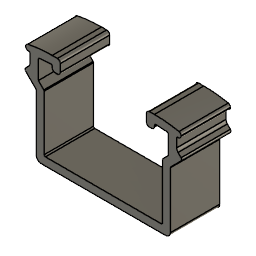
AdaptadorCristal9mm (Autodesk Fusion 360 design; units mm, degrees)
part number: 2025-12-28-14-56-03-854
Autodesk Fusion 360 part; units mm, degrees
sketch "Boceto1" plane through (0, 0, 0) normal (0, 1, 0) x (1, 0, 0)
  line L0 (2.05, 0) -> (0, 0) construction
  line L1 (3.05, 0) -> (15.65, 0)
  line L2 (2.05, -12.3964) -> (2.05, -1)
  arc A0 (3.05, 0) -> (2.05, -1) centre (3.05, -1) ccw
  line L3 (3.6762, -10.8738) -> (3.6762, -1.8762)
  line L4 (3.9262, -1.6262) -> (15.65, -1.6262)
  arc A1 (3.9262, -1.6262) -> (3.6762, -1.8762) centre (3.9262, -1.8762) ccw
  line L5 (1.9767, -12.5732) -> (-0.0927, -14.6402)
  line L6 (0.5221, -15.8217) -> (-0.093, -15.2059)
  arc A2 (-0.0927, -14.6402) -> (-0.093, -15.2059) centre (0.19, -14.9232) ccw
  line L7 (0.8, -16.4931) -> (0.8, -18.25)
  line L8 (0.6, -18.45) -> (0.45, -18.45)
  arc A3 (0.8, -16.4931) -> (0.5221, -15.8217) centre (-0.15, -16.4931) ccw
  arc A4 (0.6, -18.45) -> (0.8, -18.25) centre (0.6, -18.25) ccw
  line L9 (3.6762, -10.8738) -> (3.6762, -13.0203)
  line L10 (2.5, -14.3) -> (3.6029, -13.1971)
  line L11 (2.5, -14.3) -> (2.5, -18.0672)
  line L12 (2.7322, -18.3166) -> (5.0322, -18.4809)
  line L13 (5.3, -18.2315) -> (5.3, -17.95)
  line L14 (5.9, -17.35) -> (6.35, -17.35)
  line L15 (6.95, -17.95) -> (6.95, -19.5)
  line L16 (6.35, -20.1) -> (5.3, -20.1)
  line L17 (-0.1, -19) -> (-0.1, -19.0559)
  arc A5 (0.3391, -19.5946) -> (5.3, -20.1) centre (5.3, 4.5) ccw
  arc A6 (-0.1, -19.0559) -> (0.3391, -19.5946) centre (0.45, -19.0559) ccw
  arc A7 (0.45, -18.45) -> (-0.1, -19) centre (0.45, -19) ccw
  arc A8 (6.35, -20.1) -> (6.95, -19.5) centre (6.35, -19.5) ccw
  arc A9 (6.95, -17.95) -> (6.35, -17.35) centre (6.35, -17.95) ccw
  arc A10 (5.9, -17.35) -> (5.3, -17.95) centre (5.9, -17.95) ccw
  arc A11 (5.0322, -18.4809) -> (5.3, -18.2315) centre (5.05, -18.2315) ccw
  arc A12 (2.5, -18.0672) -> (2.7322, -18.3166) centre (2.75, -18.0672) ccw
  arc A13 (3.6029, -13.1971) -> (3.6762, -13.0203) centre (3.4262, -13.0203) ccw
  arc A14 (1.9767, -12.5732) -> (2.05, -12.3964) centre (1.8, -12.3964) ccw
  line L18 (15.65, 0) -> (15.65, -24.4844) construction
  line L19 (28.8, -14.3) -> (27.6971, -13.1971)
  line L20 (27.6238, -10.8738) -> (27.6238, -13.0203)
  arc A15 (24.35, -19.5) -> (24.95, -20.1) centre (24.95, -19.5) ccw
  line L21 (30.7, -18.45) -> (30.85, -18.45)
  line L22 (29.25, -12.3964) -> (29.25, -1)
  line L23 (26, -18.2315) -> (26, -17.95)
  line L24 (28.8, -14.3) -> (28.8, -18.0672)
  line L25 (30.7779, -15.8217) -> (31.393, -15.2059)
  arc A16 (30.5, -18.25) -> (30.7, -18.45) centre (30.7, -18.25) ccw
  line L26 (31.4, -19) -> (31.4, -19.0559)
  arc A17 (31.4, -19) -> (30.85, -18.45) centre (30.85, -19) ccw
  arc A18 (29.25, -1) -> (28.25, 0) centre (28.25, -1) ccw
  arc A19 (31.393, -15.2059) -> (31.3927, -14.6402) centre (31.11, -14.9232) ccw
  line L27 (25.4, -17.35) -> (24.95, -17.35)
  line L28 (29.3233, -12.5732) -> (31.3927, -14.6402)
  arc A20 (24.95, -17.35) -> (24.35, -17.95) centre (24.95, -17.95) ccw
  arc A21 (29.25, -12.3964) -> (29.3233, -12.5732) centre (29.5, -12.3964) ccw
  arc A22 (30.9609, -19.5946) -> (31.4, -19.0559) centre (30.85, -19.0559) ccw
  arc A23 (26, -18.2315) -> (26.2678, -18.4809) centre (26.25, -18.2315) ccw
  line L29 (29.25, 0) -> (31.3, 0) construction
  arc A24 (26, -20.1) -> (30.9609, -19.5946) centre (26, 4.5) ccw
  line L30 (24.35, -17.95) -> (24.35, -19.5)
  line L31 (24.95, -20.1) -> (26, -20.1)
  arc A25 (27.6238, -1.8762) -> (27.3738, -1.6262) centre (27.3738, -1.8762) ccw
  arc A26 (26, -17.95) -> (25.4, -17.35) centre (25.4, -17.95) ccw
  line L32 (30.5, -16.4931) -> (30.5, -18.25)
  arc A27 (28.5678, -18.3166) -> (28.8, -18.0672) centre (28.55, -18.0672) ccw
  line L33 (28.5678, -18.3166) -> (26.2678, -18.4809)
  line L34 (27.6238, -10.8738) -> (27.6238, -1.8762)
  arc A28 (30.7779, -15.8217) -> (30.5, -16.4931) centre (31.45, -16.4931) ccw
  arc A29 (27.6238, -13.0203) -> (27.6971, -13.1971) centre (27.8738, -13.0203) ccw
  line L35 (27.3738, -1.6262) -> (15.65, -1.6262)
  line L36 (28.25, 0) -> (15.65, 0)
  point P0 (31.3, 0)
  dimension "d1" = 1
  dimension "d3" = 0.25
  dimension "d4" = 0.4
  dimension "d5" = 0.95
  dimension "d6" = 0.2
  dimension "d7" = 0.55
  dimension "d8" = 0.6
  dimension "d9" = 0.25
  constraint coincident L0.end origin
  constraint horizontal L1
  constraint vertical L2
  constraint coincident L0.start L2
  constraint coincident L0.start L1
  constraint tangent L2 A0
  constraint tangent L1 A0
  constraint tangent L3 A1
  constraint tangent L4 A1
  constraint perpendicular L5 L6
  constraint tangent L5 A2
  constraint tangent L6 A2
  constraint vertical L7
  constraint perpendicular L7 L8
  constraint tangent L6 A3
  constraint tangent L7 A3
  constraint tangent L7 A4
  constraint tangent L8 A4
  constraint parallel L3 L9
  constraint parallel L7 L11
  constraint vertical L13
  constraint perpendicular L13 L14
  constraint perpendicular L14 L15
  constraint perpendicular L15 L16
  constraint perpendicular L8 L17
  constraint tangent L16 A5
  constraint tangent L17 A6
  constraint tangent A5 A6
  constraint tangent L8 A7
  constraint tangent L17 A7
  constraint equal A6 A7
  constraint tangent L15 A8
  constraint tangent L16 A8
  constraint tangent L14 A9
  constraint tangent L15 A9
  constraint equal A8 A9
  constraint tangent L13 A10
  constraint tangent L14 A10
  constraint equal A8 A10
  constraint tangent L12 A11
  constraint tangent L13 A11
  constraint tangent L11 A12
  constraint tangent L12 A12
  constraint equal A11 A12
  constraint tangent L9 A13
  constraint tangent L10 A13
  constraint equal A11 A13
  constraint tangent L2 A14
  constraint tangent L5 A14
  constraint equal A11 A14
  constraint perpendicular L4 L18
  constraint coincident L18 L4.end
  constraint symmetric L0.end L18 L29.end
  constraint symmetric L0.start L18 L29.start
  constraint symmetric L0.end L18 P0
  constraint symmetric L2.end L18 L22.end
  constraint symmetric L1.start L18 A18.end
  constraint symmetric A0 L18 A18
  constraint symmetric L3.start L18 L20.start
  constraint symmetric L3.end L18 A25.start
  constraint symmetric L4.start L18 A25.end
  constraint symmetric A1 L18 A25
  constraint symmetric L5.end L18 A19.end
  constraint symmetric L6.end L18 L25.end
  constraint symmetric A2 L18 A19
  constraint symmetric L6.start L18 L25.start
  constraint symmetric L7.start L18 L32.start
  constraint symmetric A3 L18 A28
  constraint symmetric L7.end L18 A16.start
  constraint symmetric L8.start L18 L21.start
  constraint symmetric A4 L18 A16
  constraint symmetric L10.start L18 L19.start
  constraint symmetric L16.end L18 A24.start
  constraint symmetric A5 L18 A24
  constraint symmetric L17.end L18 L26.end
  constraint symmetric A5.start L18 A22.start
  constraint symmetric A6 L18 A22
  constraint symmetric L8.end L18 L21.end
  constraint symmetric L17.start L18 L26.start
  constraint symmetric A7 L18 A17
  constraint symmetric L15.end L18 A15.start
  constraint symmetric L16.start L18 A15.end
  constraint symmetric A8 L18 A15
  constraint symmetric L14.end L18 L27.end
  constraint symmetric L15.start L18 A20.end
  constraint symmetric A9 L18 A20
  constraint symmetric L13.end L18 L23.end
  constraint symmetric L14.start L18 L27.start
  constraint symmetric A10 L18 A26
  constraint symmetric L12.end L18 A23.end
  constraint symmetric L13.start L18 L23.start
  constraint symmetric A11 L18 A23
  constraint symmetric L11.end L18 L24.end
  constraint symmetric L12.start L18 A27.start
  constraint symmetric A12 L18 A27
  constraint symmetric L9.end L18 L20.end
  constraint symmetric L10.end L18 L19.end
  constraint symmetric A13 L18 A29
  constraint symmetric L2.start L18 L22.start
  constraint symmetric L5.start L18 L28.start
  constraint symmetric A14 L18 A21
  constraint symmetric L1.end L18 L36.end
  constraint symmetric L18 L4.end L35.end
  measures "d1" radius of A0
  measures "d3" radius of A1
  measures "d4" radius of A2
  measures "d5" radius of A3
  measures "d6" radius of A4
  measures "d7" radius of A6
  measures "d8" radius of A8
  measures "d9" radius of A11
extrude "Extruir1" add sketch "Boceto1" along normal blind 10
equation "L = 10 mm"
equation "d11 = L"
